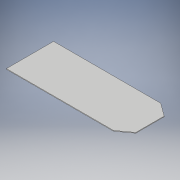
# Autodesk Inventor part: 140x55mm-PCB
Saved by Autodesk Inventor 2018 (Build 220112000, 112)
## iProperties
Created: 2018-04-06
Part Number: 140x55mm-PCB
Material: Generic
Document SubType Name: Modeling
Designer: bbramman
Density: 1 g/cm^3
Appearance: Default
Author: bbramman
Autodesk Inventor part; units mm, degrees
ref_plane "YZ Plane" through (0, 0, 0) normal (1, 0, 0) x (0, 1, 0)
ref_plane "XZ Plane" through (0, 0, 0) normal (0, 1, 0) x (-1, 0, 0)
ref_plane "XY Plane" through (0, 0, 0) normal (0, 0, 1) x (1, 0, 0)
sketch "Sketch1" plane through (0, 0, 0) normal (0, 1, 0) x (-1, 0, 0)
  line L0 (-62.5, 27.5) -> (62.5, 27.5)
  line L1 (62.5, 27.5) -> (62.5, -27.5)
  line L2 (62.5, -27.5) -> (-62.5, -27.5)
  line L3 (-62.5, 27.5) -> (62.5, -27.5) construction
  line L4 (62.5, 27.5) -> (-62.5, -27.5) construction
  line L5 (-77.4954, -16.5) -> (-77.4954, 16.5)
  line L6 (-77.4954, -16.5) -> (-44.4954, -16.5) construction
  line L7 (-62.5, 27.5) -> (-77.4954, 16.5)
  line L8 (-77.4954, -16.5) -> (-62.5, -27.5)
  point P0 (0, 0)
  dimension "d0" = 125
  dimension "d1" = 55
  dimension "d2" = 33
  dimension "d3" = 90
  constraints: 18 end point, 2 horizontal, 2 midpoint, 2 perpendicular, 1 parallel
  measures "d0" distance of L1.end L2.end
  measures "d1" distance of L0.end L1.end
  measures "d2" distance of L5.start L5.end
  measures "d3" angle of L6 L5
extrude "Extrusion1" add sketch "Sketch1" along normal mid plane 0.7874
body "Solid1"
